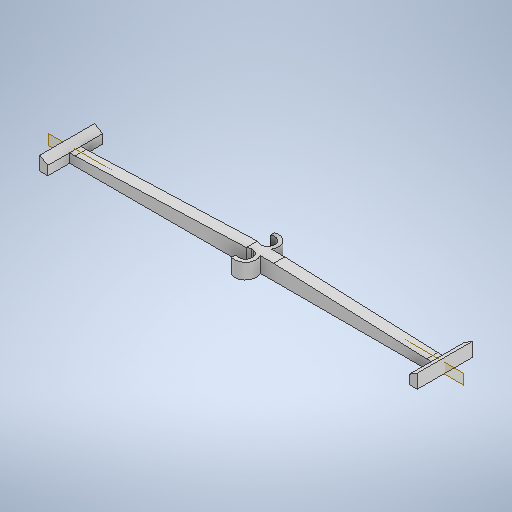
# Autodesk Inventor part: 2025_08_29_Holder_2NMR_tubes
Saved by Autodesk Inventor 2025.1 (Build 291241000, 241)
## iProperties
Created: 2024-08-23
Part Number: 2025_08_29_Holder_2NMR_tubes
Material: Generisch
Document SubType Name: Modeling
Designer: to86hug
Density: 1 g/cm^3
Appearance: Vorgabe
Author: to86hug
Autodesk Inventor part; units mm, degrees
ref_plane "YZ Plane" through (0, 0, 0) normal (1, 0, 0) x (0, 1, 0)
ref_plane "XZ Plane" through (0, 0, 0) normal (0, 1, 0) x (-1, 0, 0)
ref_plane "XY Plane" through (0, 0, 0) normal (0, 0, 1) x (1, 0, 0)
sketch "Skizze1" plane through (0, 0, 0) normal (0, 0, 1) x (1, 0, 0)
  line L0 (-68.016, 1.808) -> (67.584, 1.808)
  line L1 (67.584, 1.808) -> (67.584, -2.192)
  line L2 (67.584, -2.192) -> (-68.016, -2.192)
  line L3 (-68.016, -2.192) -> (-68.016, 1.808)
  line L4 (-68.016, 1.808) -> (67.584, -2.192) construction
  line L5 (67.584, 1.808) -> (-68.016, -2.192) construction
  point P0 (0, 0)
  point P1 (-0.216, -0.192)
  point P2 (-0.216, -0.192)
  dimension "d0" = 135.6
  dimension "d1" = 4
  constraints: 12 end point, 2 midpoint, 2 parallel, 1 horizontal, 1 perpendicular
  measures "d0" distance of L0.start L0.end
  measures "d1" distance of L0.end L1.end
extrude "Extrusion1" add sketch "Skizze1" along normal mid plane 3.25
ref_plane "Arbeitsebene1" through (-68.016, -0.192, 1.625) normal (0, -1, 0) x (1, 0, 0)
sketch "Skizze2" plane through (-68.016, -0.192, 1.625) normal (0, -1, 0) x (1, 0, 0)
  line L0 (0, -3.25) -> (0, 0) projected
  line L1 (0, -3.25) -> (135.6, -3.25) projected
  line L2 (0, 0) -> (2.85, 0)
  line L3 (2.85, 0) -> (2.85, -3.25)
  line L4 (2.85, -3.25) -> (0, -3.25)
  line L5 (0, -3.25) -> (0, 0)
  line L6 (0, 0) -> (0, 1.75)
  line L7 (0, 1.75) -> (2.85, 0)
  line L8 (135.6, -3.25) -> (135.6, 0) projected
  line L9 (135.6, 0) -> (132.75, 0)
  line L10 (132.75, 0) -> (132.75, -3.25)
  line L11 (132.75, -3.25) -> (135.6, -3.25)
  line L12 (135.6, -3.25) -> (135.6, 0)
  line L13 (135.6, 0) -> (135.6, 1.75)
  line L14 (135.6, 1.75) -> (132.75, 0)
  point P0 (68.016, -1.625)
  dimension "d4" = 2.85
  dimension "d5" = 1.75
  dimension "d6" = 2.85
  constraints: 24 end point, 4 parallel, 2 horizontal, 2 perpendicular, 2 point on line, 2 vertical
  measures "d4" distance of L3.end L4.end
  measures "d5" distance of L0.end L6.end
  measures "d6" distance of L11.end L10.end
extrude "Extrusion2" add sketch "Skizze2" along normal mid plane 19.7
sketch "Skizze5" plane through (0, 0, 1.625) normal (0, 0, 1) x (1, 0, 0)
  line L0 (64.734, 1.808) -> (-65.166, 1.808) projected
  line L1 (64.734, -2.192) -> (-65.166, -2.192) projected
  line L2 (-1.7094, 1.808) -> (-63.2094, 1.808)
  line L3 (-63.2094, 1.808) -> (-63.2094, -2.192)
  line L4 (-63.2094, -2.192) -> (-1.7094, -2.192)
  line L5 (-1.7094, -2.192) -> (-1.7094, 1.808)
  line L6 (-65.166, -2.192) -> (64.734, -2.192) projected
  line L7 (3.1164, 1.808) -> (63.1164, 1.808)
  line L8 (63.1164, 1.808) -> (63.1164, -2.192)
  line L9 (63.1164, -2.192) -> (3.1164, -2.192)
  line L10 (3.1164, -2.192) -> (3.1164, 1.808)
  point P0 (0, 0)
  point P1 (-8.6889, 1.808)
  point P2 (-8.6001, -2.192)
  point P3 (8.6889, 1.808)
  point P4 (8.6001, -2.192)
  point P5 (3.1164, -2.192)
  point P6 (-1.7094, -2.192)
  point P7 (-63.2094, 1.808)
  point P8 (3.1164, -2.192)
  point P9 (63.1164, -2.192)
  point P10 (-1.7094, 1.808)
  point P11 (-1.7094, -2.192)
  point P12 (-3.4528, 1.808)
  point P13 (-3.2227, -2.192)
  point P14 (3.2227, -2.192)
  point P15 (-4.9028, 1.808)
  dimension "d17" = 61.5
  dimension "d18" = 60
  constraints: 16 end point, 4 parallel, 2 horizontal, 2 perpendicular
  measures "d17" distance of L4.end L3.end
  measures "d18" distance of L8.end L9.end
extrude "Extrusion5" add sketch "Skizze5" along normal blind 2.25 contours L8 L1 L10 L0 | L5 L1 L3 L0
sketch "Skizze6" plane through (-65.166, -2.192, -1.625) normal (0, -1, 0) x (1, 0, 0)
  line L0 (1.9566, 5.5) -> (63.4566, 5.5) projected
  line L1 (1.9566, 5.5) -> (63.4566, 5.5)
  line L2 (56.9566, 5.5) -> (56.9566, 3.25)
  line L3 (56.9566, 3.25) -> (1.9566, 3.25)
  line L4 (1.9566, 3.25) -> (1.9566, 5.5)
  line L5 (63.4566, 5.5) -> (1.9566, 3.25)
  line L6 (128.2824, 3.25) -> (128.2824, 5.5) projected
  line L7 (128.2824, 5.5) -> (73.2824, 5.5)
  line L8 (73.2824, 5.5) -> (73.2824, 3.25)
  line L9 (73.2824, 3.25) -> (128.2824, 3.25)
  line L10 (128.2824, 3.25) -> (128.2824, 5.5)
  line L11 (73.2824, 5.5) -> (128.2824, 3.25)
  point P0 (65.166, 1.625)
  point P1 (56.5659, 5.5)
  point P2 (56.5659, 5.5)
  point P3 (56.5659, 5.5)
  dimension "d21" = 55
  dimension "d22" = 2.25
  dimension "d23" = 55
  dimension "d26" = 2.25
  constraints: 20 end point, 4 parallel, 2 horizontal, 2 perpendicular
  measures "d21" distance of L2.end L3.end
  measures "d22" vertical distance of L0.end L2.end
  measures "d23" distance of L9.end L8.end
  measures "d26" distance of L7.end L8.end
extrude "Extrusion6" cut sketch "Skizze6" against normal through all contours L0 L2 L5 L4 | L0 L5 L2 | L11 L7 L6
sketch "Skizze7" plane through (0, 0, -1.625) normal (0, 0, -1) x (-1, 0, 0)
  line L0 (0, 0) -> (0, -0.192) construction
  line L1 (0, -0.192) -> (0, -4.192) construction
  line L2 (0, -0.192) -> (0, 3.808) construction
  circle A0 centre (0, -4.192) radius 2.55
  circle A1 centre (0, -4.192) radius 3.9
  circle A2 centre (0, 3.808) radius 3.9
  circle A3 centre (0, 3.808) radius 2.55
  line L3 (1.2597, -9.2691) -> (1.2597, 9.3057)
  point P0 (1.2597, 6.0252)
  point P1 (1.2597, 7.499)
  point P2 (1.2597, 0.1171)
  point P3 (1.2597, 1.5909)
  point P4 (1.2597, -1.9748)
  point P5 (1.2597, -0.501)
  point P6 (1.2597, -7.8829)
  point P7 (1.2597, -6.4091)
  dimension "d30" = 4
  dimension "d31" = 4
  dimension "d32" = 5.1
  dimension "d34" = 7.8
  dimension "d35" = 7.8
  dimension "d36" = 5.1
  constraints: 8 end point, 4 centre point, 4 coincident, 3 vertical, 1 point on line
  measures "d30" distance of L0.end L1.end
  measures "d31" distance of L0.end L2.end
  measures "d32" diameter of A0
  measures "d34" diameter of A1
  measures "d35" diameter of A2
  measures "d36" diameter of A3
extrude "Extrusion8" add sketch "Skizze7" against normal blind 5.5 contours A0 L3 A1 | L3 A3 A2 picked at (0.7662, -0.8482) picked at (0.7662, 7.1518)
sketch "Skizze9" plane through (0, 0, 3.875) normal (0, 0, 1) x (1, 0, 0)
  arc A0 (1.5819, -2.192) -> (-1.2597, -1.9748) centre (0, -4.192) ccw construction
  circle A1 centre (0, -4.192) radius 2.55
  arc A2 (-1.2597, 1.5909) -> (-1.2597, 6.0252) centre (0, 3.808) ccw construction
  circle A3 centre (0, 3.808) radius 2.55
  line L0 (0, 1.258) -> (-1.7094, 1.258)
  line L1 (-1.7094, 1.808) -> (-1.7094, -2.192) projected
  line L2 (3.1164, -1.8472) -> (3.1164, 1.4633) projected
  line L3 (-1.7094, 1.258) -> (3.1164, 1.258)
  line L4 (3.1164, 1.258) -> (3.1164, -1.642) construction
  line L5 (3.1164, -1.642) -> (-1.7094, -1.642)
  line L6 (-1.7094, -1.642) -> (-1.7094, 1.258) construction
  point P0 (0, 0)
  dimension "d41" = 5.1
  constraints: 10 end point, 2 coincident, 2 horizontal, 2 parallel, 2 point on line, 1 centre point, 1 perpendicular, 1 vertical alignment, 2 other
extrude "Extrusion9" cut sketch "Skizze9" against normal through all contours A1 | A3
sketch "Skizze10" plane through (0, 0, 3.875) normal (0, 0, 1) x (1, 0, 0)
  arc A0 (-1.2597, 1.5909) -> (-1.2597, 6.0252) centre (0, 3.808) ccw construction
  line L0 (0, 1.258) -> (-1.7094, 1.258) construction
  line L1 (-1.7094, 1.808) -> (-1.7094, -2.192) construction
  line L2 (3.1164, 1.4633) -> (3.1164, -1.8472) projected
  line L3 (-1.7094, 1.258) -> (3.1164, 1.258)
  line L4 (3.1164, 1.258) -> (3.1164, -1.6642)
  line L5 (3.1164, -1.6642) -> (-1.7094, -1.6642)
  line L6 (-1.7094, -1.6642) -> (-1.7094, 1.258)
  line L7 (2.9224, 1.258) -> (3.4334, 1.258)
  line L8 (3.4334, 1.258) -> (3.4334, 1.5422)
  line L9 (3.4334, 1.5422) -> (2.9224, 1.5422)
  line L10 (2.9224, 1.5422) -> (2.9224, 1.258)
  line L11 (2.9224, -1.6642) -> (3.3541, -1.6642)
  line L12 (3.3541, -1.6642) -> (3.3541, -1.947)
  line L13 (3.3541, -1.947) -> (2.9224, -1.947)
  line L14 (2.9224, -1.947) -> (2.9224, -1.6642)
  point P0 (0, 0)
  constraints: 26 end point, 6 parallel, 5 point on line, 4 horizontal, 3 perpendicular, 1 point on circle
extrude "Extrusion10" add sketch "Skizze10" against normal blind 5.5
sketch "Skizze11" plane through (0, 0, 3.875) normal (0, 0, 1) x (1, 0, 0)
  line L0 (-1.2597, 1.258) -> (-1.2597, 1.5909) projected
  line L1 (-1.2597, 1.5909) -> (-1.2597, 1.258)
  line L2 (-1.7094, -1.6642) -> (-1.7094, 1.258) projected
  line L3 (-1.2597, 1.258) -> (-1.7094, 1.258)
  line L4 (-1.7094, 1.258) -> (-1.7094, 1.8077)
  line L5 (-1.7094, 1.8077) -> (-1.5839, 1.8077)
  arc A0 (-1.5839, 1.8077) -> (-1.2597, 1.5909) centre (0.106, 3.9847) ccw
  line L6 (-1.5819, -2.192) -> (-65.166, -2.192) projected
  arc A1 (-0.3356, -1.6642) -> (-1.5819, -2.192) centre (0, -4.192) ccw projected
  line L7 (-1.2597, -1.6642) -> (-1.2597, -1.9748) projected
  arc A2 (-1.5819, -2.192) -> (-1.41, -2.0673) centre (0, -4.192) ccw
  line L8 (-1.2597, -1.9748) -> (-1.2597, -1.6642)
  line L9 (-1.2597, -1.6642) -> (-1.7094, -1.6642) projected
  line L10 (-1.7094, -1.6642) -> (-1.7094, -2.192) projected
  line L11 (-1.7094, -1.6642) -> (-1.7094, -2.192)
  line L12 (-1.7094, -2.192) -> (-1.5819, -2.192)
  point P0 (0, 0)
  constraints: 14 end point, 6 point on circle, 4 perpendicular, 2 centre point, 2 collinear, 1 vertical
extrude "Extrusion11" add sketch "Skizze11" against normal blind 5.5 contours L3 L4 L5 A0 L0 | L6 L10 L9 L7 A1
